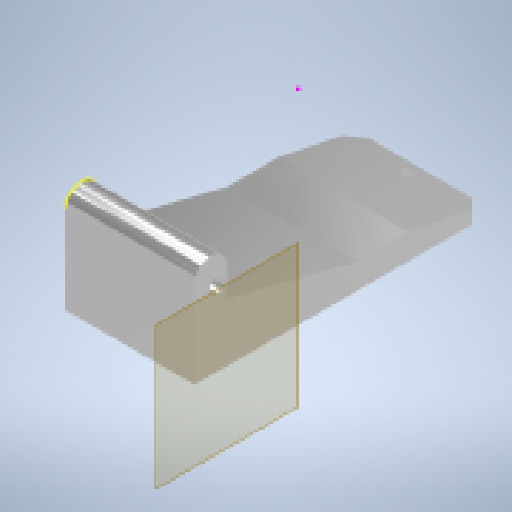
# Autodesk Inventor part: Bremse
Saved by Autodesk Inventor 2025 (Build 290162010, 162A)
## iProperties
Created: 2024-11-26
Part Number: Bremse
Material: Aluminium 6061(1)
Document SubType Name: Modeling
Designer: Admin
Density: 2.7 g/cm^3
Appearance: Aluminium - flach(1)
Author: Admin
Autodesk Inventor part; units mm, degrees
ref_plane "YZ Plane" through (0, 0, 0) normal (1, 0, 0) x (0, 1, 0)
ref_plane "XZ Plane" through (0, 0, 0) normal (0, 1, 0) x (-1, 0, 0)
ref_plane "XY Plane" through (0, 0, 0) normal (0, 0, 1) x (1, 0, 0)
sketch "Skizze1" plane through (0, 0, 0) normal (0, 0, 1) x (1, 0, 0)
  line L0 (15.26, -39.0647) -> (-4.74, -39.0647)
  line L1 (-4.74, -39.0647) -> (-4.74, 5.9353)
  line L2 (-4.74, 5.9353) -> (15.26, 5.9353)
  line L3 (15.26, 5.9353) -> (15.26, -39.0647)
  dimension "d2" = 20
  dimension "d3" = 45
  constraints: 8 end point, 2 parallel, 1 horizontal, 1 perpendicular
  measures "d2" distance of L1.end L2.end
  measures "d3" distance of L0.end L1.end
extrude "Extrusion1" add sketch "Skizze1" along normal blind 4
sketch "Skizze3" plane through (0, 0, 4) normal (0, 0, 1) x (1, 0, 0)
  line L0 (15.26, -39.0647) -> (-4.74, -39.0647)
  line L1 (-4.74, 5.9353) -> (-4.74, -39.0647) projected
  line L2 (15.26, -39.0647) -> (-4.74, -39.0647)
  line L3 (-4.74, -39.0647) -> (-4.74, -34.0647)
  line L4 (-4.74, -34.0647) -> (15.26, -34.0647)
  line L5 (15.26, -34.0647) -> (15.26, -39.0647)
  line L6 (-4.74, -39.0647) -> (15.26, -39.0647) projected
  point P0 (0, 0)
  point P1 (15.26, -34.0647)
  point P2 (15.26, -34.0647)
  point P3 (15.26, -34.0647)
  dimension "d8" = 5
  constraints: 6 end point, 2 horizontal, 1 parallel, 1 point on line, 1 vertical, 6 other
  measures "d8" distance of L3.start L3.end
extrude "Extrusion3" add sketch "Skizze3" along normal blind 12
fillet "Rundung2" radius 2.5 2 edges at (5.26, -34.0647, 16) (5.26, -39.0647, 16)
sketch "Skizze4" plane through (-4.74, 5.9353, 0) normal (-1, 0, 0) x (0, 0, 1)
  arc A0 (13.5, -45) -> (13.5, -40) centre (13.5, -42.5) ccw projected
  point P0 (0, -5.9353)
  point P1 (11.5901, -9.0016)
  point P2 (11.5, -40)
hole "Bohrung1" at (-4.74, -36.5647, 13.5) direction (1, 0, 0) diameter 2.2 depth 5 tip angle 118
chamfer "Fasen2" distance 2 angle 45 2 edges at (-4.74, 5.9353, 2) (15.26, 5.9353, 2)
chamfer "Fasen3" distance 5 distance2 20 1 edges at (5.26, -34.0647, 4) measured on face at (5.26, -34.0647, 4.5)
ref_plane "Arbeitsebene1" through (15.26, -34.0647, 0) normal (1, 0, 0) x (0, 0, -1)
sketch "Skizze7" plane through (15.26, -34.0647, 0) normal (1, 0, 0) x (0, 0, -1)
  circle A0 centre (-13.5, -2.5) radius 1.1 projected
  point P0 (0, 34.0647)
  constraints: 1 coincident
hole "Bohrung3" at (15.26, -36.5647, 13.5) direction (-1, 0, 0) diameter 2.2 depth 5 tip angle 118
chamfer "Fasen5" distance 12 distance2 2.5 1 edges at (5.26, 5.9353, 4) measured on face at (5.26, 5.4353, 4)
sketch "Skizze8" plane through (0, 0, 0) normal (0, 0, -1) x (-1, 0, 0)
  line L0 (-13.26, 5.9353) -> (2.74, 5.9353) construction
  line L1 (-5.26, 3.9353) -> (-5.26, 5.9353) construction
  point P0 (0, 0)
  dimension "d53" = 2
  constraints: 2 end point, 1 midpoint, 1 perpendicular
  measures "d53" distance of L1.end L1.start
hole "Bohrung4" at (5.26, 3.9353, 0) direction (0, 0, 1) diameter 2 end through all
chamfer "Fasen6" distance 1 distance2 12 1 edges at (5.26, 5.9353, 0) measured on face at (5.26, 5.9353, 0.5)
thicken "Verdickung1" operation add thickness 2 both sides no extend neighbours no toward (0, 0, 1) faces at (1.9266, -8.7314, 4)
chamfer "Fasen7" distance 20 distance2 2 1 edges at (-4.74, -10.0647, 6) measured on face at (-4.24, -10.0647, 6)
chamfer "Fasen8" distance 20 distance2 2 1 edges at (5.26, -39.0647, 0) measured on face at (5.26, -38.5647, 0)
fillet "Rundung4" radius 2 1 edges at (5.26, -39.0647, 2)
